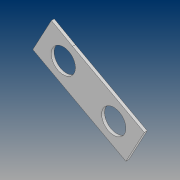
# Autodesk Inventor part: asfaleia_koxlia
Saved by Autodesk Inventor 2021 (Build 250183000, 183)
## iProperties
Created: 2021-01-09
Part Number: asfaleia_koxlia
Material: Generic
Document SubType Name: Modeling
Designer: Angelos
Density: 1 g/cm^3
Appearance: Default
Author: Angelos
Autodesk Inventor part; units mm, degrees
ref_plane "YZ Plane" through (0, 0, 0) normal (1, 0, 0) x (0, 1, 0)
ref_plane "XZ Plane" through (0, 0, 0) normal (0, 1, 0) x (-1, 0, 0)
ref_plane "XY Plane" through (0, 0, 0) normal (0, 0, 1) x (1, 0, 0)
sketch "Sketch1" plane through (0, 0, 0) normal (0, 0, 1) x (1, 0, 0)
  circle A0 centre (105.4319, 133.3571) radius 12.5
  circle A1 centre (53.4628, 161.3745) radius 12.5
  line L0 (53.4628, 161.3745) -> (105.4319, 133.3571)
  line L1 (105.4319, 133.3571) -> (114.9229, 150.9617)
  line L2 (53.4628, 161.3745) -> (62.9538, 178.9791)
  line L3 (62.9538, 178.9791) -> (114.9229, 150.9617)
  line L4 (114.9229, 150.9617) -> (136.9286, 139.098)
  line L5 (136.9286, 139.098) -> (117.9468, 103.8888)
  line L6 (117.9468, 103.8888) -> (21.9682, 155.6324)
  line L7 (21.9682, 155.6324) -> (41.1135, 191.1447)
  line L8 (62.9538, 178.9791) -> (41.1135, 191.1447)
  point P0 (0, 0)
  point P1 (0, 0)
  dimension "d25" = 25
  dimension "d26" = 170
  dimension "d27" = 25
  dimension "d38" = 161.3745
  dimension "d39" = 53.4628
  dimension "d40" = 105.4319
  dimension "d41" = 133.3571
  dimension "d43" = 90
  dimension "d44" = 90
  dimension "d46" = 20
  dimension "d47" = 20
  dimension "d48" = 25
  dimension "d49" = 40
  dimension "d50" = 90
  dimension "d51" = 90
  dimension "d52" = 90
  dimension "d54" = 25
  constraints: 18 end point, 2 centre point, 1 perpendicular
  measures "d25" diameter of A1
  measures "d26" distance of L0.start point (0, 0)
  measures "d27" diameter of A0
  measures "d38" vertical distance of point (0, 0) L0.start
  measures "d39" horizontal distance of point (0, 0) L0.start
  measures "d40" horizontal distance of point (0, 0) L0.end
  measures "d41" vertical distance of point (0, 0) L0.end
  measures "d43" angle of L1 L0
  measures "d44" angle of L0 L2
  measures "d46" distance of L0.start L2.end
  measures "d47" distance of L0.end L1.end
  measures "d48" distance of L1.end L4.end
  measures "d49" distance of L4.end L5.end
  measures "d50" angle of L4 L5
  measures "d51" angle of L5 L6
  measures "d52" angle of L6 L7
  measures "d54" distance of L7.end L2.end
extrude "Extrusion1" add sketch "Sketch1" along normal blind 3 contours A0 L1 L4 L5 L6 L7 L8 L2 A1 L0 | A0 L0 A1 L2 L3 L1
body "Solid1"
